gear-pinion v8 (Autodesk Fusion 360 design; units mm, degrees)
description: Spur Gear; Module: 0.4; Num Teeth: 7; Pressure Angle: 20.0; Backlash: 0.01 mm
description: Spur Gear; Module: 0.4; Num Teeth: 7; Pressure Angle: 20.0; Backlash: 0.00 mm
Autodesk Fusion 360 part; units mm, degrees
sketch "スケッチ1" plane through (0, 0, 0) normal (0, 0, 1) x (1, 0, 0) in component "Spur Gear (7 teeth)"
  circle A0 centre (0, 0) radius 0.8692
  circle A1 centre (0, 0) radius 0.25
extrude "押し出し1" add sketch "スケッチ1" along normal blind 2 makes body 1 in component "Spur Gear (7 teeth)"
sketch "スケッチ2" plane through (0, 0, 0) normal (0, 0, 1) x (1, 0, 0) in component "Spur Gear (7 teeth)"
  spline S0 degree 3 poles (1.2786, -0.3095) (1.2969, -0.311) (1.3342, -0.314) (1.391, -0.306) (1.4488, -0.2928) (1.5073, -0.2734) (1.5661, -0.2487) (1.6249, -0.2188) (1.6834, -0.1837) (1.7414, -0.1439) (1.7785, -0.1139) (1.7973, -0.0987) knots 0 0 0 0 0.00548 0.011189 0.01712 0.023272 0.029644 0.036236 0.043049 0.050082 0.057335 0.057335 0.057335 0.057335
  spline S1 degree 3 poles (1.2786, 0.3095) (1.2969, 0.311) (1.3342, 0.314) (1.391, 0.306) (1.4488, 0.2928) (1.5073, 0.2734) (1.5661, 0.2487) (1.6249, 0.2188) (1.6834, 0.1837) (1.7414, 0.1439) (1.7785, 0.1139) (1.7973, 0.0987) knots 0 0 0 0 0.00548 0.011189 0.01712 0.023272 0.029644 0.036236 0.043049 0.050082 0.057335 0.057335 0.057335 0.057335
  arc A0 (1.7973, -0.0987) -> (1.7973, 0.0987) centre (0, 0) ccw
  line L0 (0.8351, -0.2045) -> (1.2786, -0.3095)
  line L1 (0.8351, 0.2045) -> (1.2786, 0.3095)
  line L2 (0.8351, -0.2045) -> (0.8351, 0.2045)
  point P0 (1.3334, -0.312)
  point P1 (1.3901, -0.3053)
  point P2 (1.4479, -0.2921)
  point P3 (1.5063, -0.2729)
  point P4 (1.5651, -0.2483)
  point P5 (1.6239, -0.2184)
  point P6 (1.6824, -0.1835)
  point P7 (1.7403, -0.1436)
  point P8 (1.3334, 0.312)
  point P9 (1.3901, 0.3053)
  point P10 (1.4479, 0.2921)
  point P11 (1.5063, 0.2729)
  point P12 (1.5651, 0.2483)
  point P13 (1.6239, 0.2184)
  point P14 (1.6824, 0.1835)
  point P15 (1.7403, 0.1436)
extrude "押し出し2" add sketch "スケッチ2" along normal blind 2 bodies 1 in component "Spur Gear (7 teeth)"
fillet "フィレット1" radius 0.21 2 edges at (0.8443, -0.2067, 1) (0.8443, 0.2067, 1) on bodies 1 in component "Spur Gear (7 teeth)"
pattern_circular "C パターン1" count 7 over 360 about axis through (0, 0, 0) along (0, 0, 1) of "押し出し2", "フィレット1" in component "Spur Gear (7 teeth)"
sketch "スケッチ3" plane through (0, 0, 0) normal (0, 0, 1) x (1, 0, 0) in component "Spur Gear (7 teeth)"
  circle A0 centre (0, 0) radius 1.4 construction
sketch "スケッチ1 (2)" plane through (0, 0, 0) normal (0, 0, 1) x (1, 0, 0) in component "Spur Gear (7 teeth) (1)"
  circle A0 centre (0, 0) radius 0.8692
  circle A1 centre (0, 0) radius 0.4
extrude "押し出し1'" add sketch "スケッチ1 (2)" along normal blind 2 separate body makes body 2 in component "Spur Gear (7 teeth) (1)"
sketch "スケッチ2 (2)" plane through (0, 0, 0) normal (0, 0, 1) x (1, 0, 0) in component "Spur Gear (7 teeth) (1)"
  spline S0 degree 3 poles (1.2781, -0.3118) (1.2963, -0.3133) (1.3336, -0.3164) (1.3905, -0.3085) (1.4483, -0.2954) (1.5068, -0.2761) (1.5657, -0.2515) (1.6245, -0.2217) (1.683, -0.1867) (1.7412, -0.147) (1.7783, -0.1171) (1.7971, -0.1019) knots 0 0 0 0 0.00548 0.011189 0.01712 0.023272 0.029644 0.036236 0.043049 0.050082 0.057335 0.057335 0.057335 0.057335
  spline S1 degree 3 poles (1.2781, 0.3118) (1.2963, 0.3133) (1.3336, 0.3164) (1.3905, 0.3085) (1.4483, 0.2954) (1.5068, 0.2761) (1.5657, 0.2515) (1.6245, 0.2217) (1.683, 0.1867) (1.7412, 0.147) (1.7783, 0.1171) (1.7971, 0.1019) knots 0 0 0 0 0.00548 0.011189 0.01712 0.023272 0.029644 0.036236 0.043049 0.050082 0.057335 0.057335 0.057335 0.057335
  arc A0 (1.7971, -0.1019) -> (1.7971, 0.1019) centre (0, 0) ccw
  line L0 (0.8347, -0.206) -> (1.2781, -0.3118)
  line L1 (0.8347, 0.206) -> (1.2781, 0.3118)
  line L2 (0.8347, -0.206) -> (0.8347, 0.206)
  point P0 (1.3328, -0.3144)
  point P1 (1.3895, -0.3078)
  point P2 (1.4474, -0.2946)
  point P3 (1.5059, -0.2756)
  point P4 (1.5647, -0.2511)
  point P5 (1.6235, -0.2213)
  point P6 (1.682, -0.1865)
  point P7 (1.74, -0.1467)
  point P8 (1.3328, 0.3144)
  point P9 (1.3895, 0.3078)
  point P10 (1.4474, 0.2946)
  point P11 (1.5059, 0.2756)
  point P12 (1.5647, 0.2511)
  point P13 (1.6235, 0.2213)
  point P14 (1.682, 0.1865)
  point P15 (1.74, 0.1467)
extrude "押し出し2'" add sketch "スケッチ2 (2)" along normal blind 2 bodies 2 in component "Spur Gear (7 teeth) (1)"
pattern_circular "C パターン1'" count 7 over 360 about axis through (0, 0, 0) along (0, 0, 1) of "押し出し2'" in component "Spur Gear (7 teeth) (1)"
sketch "スケッチ3 (2)" plane through (0, 0, 0) normal (0, 0, 1) x (1, 0, 0) in component "Spur Gear (7 teeth) (1)"
  circle A0 centre (0, 0) radius 1.4 construction
component "Spur Gear (7 teeth) (1)" placed x (1, 0, 0) y (0, 1, 0) z (0, 0, 1) at (0, 0, 0)
